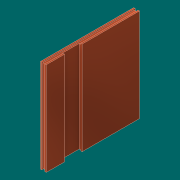
# Autodesk Inventor part: sides
Saved by Autodesk Inventor 2016 (Build 200138000, 138)
## iProperties
Created: 2015-10-13
Part Number: sides
Material: PC/ABS Plastic
Document SubType Name: Modeling
Designer: Sawaiz
Density: 0.357273 g/cm^3
Appearance: Copper - Polished
Author: Sawaiz
Autodesk Inventor part; units mm, degrees
ref_plane "YZ Plane" through (0, 0, 0) normal (1, 0, 0) x (0, 1, 0)
ref_plane "XZ Plane" through (0, 0, 0) normal (0, 1, 0) x (-1, 0, 0)
ref_plane "XY Plane" through (0, 0, 0) normal (0, 0, 1) x (1, 0, 0)
sketch "Sketch1" plane through (0, 0, 0) normal (0, 1, 0) x (-1, 0, 0)
  line L0 (-50.8, 50.8) -> (50.8, 50.8)
  line L1 (50.8, 50.8) -> (50.8, -50.8)
  line L2 (50.8, -50.8) -> (-50.8, -50.8)
  line L3 (-50.8, -50.8) -> (-50.8, 50.8)
  line L4 (-50.8, 50.8) -> (50.8, -50.8) construction
  line L5 (50.8, 50.8) -> (-50.8, -50.8) construction
  point P0 (0, 0)
  dimension "d0" = 101.6
  dimension "d1" = 101.6
  constraints: 12 end point, 2 midpoint, 2 parallel, 1 horizontal, 1 perpendicular
  measures "d0" distance of L1.end L2.end
  measures "d1" distance of L0.end L1.end
extrude "Extrusion1" add sketch "Sketch1" along normal blind 6.35
sketch "Sketch2" plane through (0, 6.35, 0) normal (0, 1, 0) x (1, 0, 0)
  line L0 (-50.8, -50.8) -> (50.8, -50.8) projected
  line L1 (50.8, -50.8) -> (50.8, 50.8) projected
  line L2 (50.8, 50.8) -> (-50.8, 50.8) projected
  line L3 (-50.8, 50.8) -> (-50.8, -50.8) projected
  line L4 (-50.8, -50.8) -> (50.8, -50.8) projected
  line L5 (30.8, 50.8) -> (11.75, 50.8)
  line L6 (11.75, 50.8) -> (11.75, -50.8)
  line L7 (11.75, -50.8) -> (30.8, -50.8)
  line L8 (30.8, -50.8) -> (30.8, 50.8)
  line L9 (30.8, 50.8) -> (11.75, -50.8) construction
  line L10 (11.75, 50.8) -> (30.8, -50.8) construction
  point P0 (0, 0)
  point P1 (21.275, 0)
  dimension "d4" = 19.05
  dimension "d5" = 20
  constraints: 12 end point, 2 collinear, 2 midpoint, 2 parallel, 1 horizontal, 1 perpendicular
  measures "d4" distance between parallel lines of L6 L8
  measures "d5" distance between parallel lines of L1 L8
extrude "Extrusion2" cut sketch "Sketch2" against normal blind 3.175 contours L6 L2 L8 L0
sketch "Sketch5" plane through (50.8, 0, 50.8) normal (1, 0, 0) x (0, 0, -1)
  line L0 (101.6, 0) -> (0, 0) projected
  line L1 (101.6, 0) -> (101.6, 6.35) projected
  line L2 (0, 6.35) -> (101.6, 6.35) projected
  line L3 (0, 0) -> (0, 6.35) projected
  line L4 (0, 0) -> (0, 6.35) projected
  line L5 (0, 3.175) -> (101.6, 3.175)
  line L6 (101.6, 1.5875) -> (0, 1.5875)
  line L7 (0, 1.5875) -> (0, 4.7625)
  line L8 (0, 4.7625) -> (101.6, 4.7625)
  line L9 (101.6, 4.7625) -> (101.6, 1.5875)
  line L10 (0, 3.175) -> (101.6, 3.175) projected
  line L11 (101.6, 1.5875) -> (0, 4.7625) construction
  line L12 (0, 1.5875) -> (101.6, 4.7625) construction
  point P0 (50.8, 0)
  point P1 (50.8, 3.175)
  point P2 (6.35, 3.175)
  point P3 (95.25, 3.175)
  dimension "d34" = 3.175
  constraints: 14 end point, 5 midpoint, 2 parallel, 1 horizontal, 1 perpendicular, 1 point on line
  measures "d34" distance between parallel lines of L8 L6
extrude "Extrusion3" cut sketch "Sketch5" against normal blind 0.9525 contours L6 L3 L5 L1 | L5 L3 L8 L1
mirror "Mirror3" about plane through (0, 0, 0) normal (1, 0, 0) of "Extrusion3"
sketch "Sketch6" plane through (-50.8, 0, 50.8) normal (0, 0, 1) x (1, 0, 0)
  line L0 (0, 4.7625) -> (0.9525, 4.7625) projected
  line L1 (0.9525, 4.7625) -> (0.9525, 1.5875) projected
  line L2 (0.9525, 1.5875) -> (0, 1.5875) projected
  line L3 (0, 0) -> (0, 1.5875) projected
  line L4 (101.6, 0) -> (0, 0) projected
  line L5 (101.6, 0) -> (101.6, 1.5875) projected
  line L6 (101.6, 1.5875) -> (100.6475, 1.5875) projected
  line L7 (100.6475, 1.5875) -> (100.6475, 4.7625) projected
  line L8 (100.6475, 4.7625) -> (101.6, 4.7625) projected
  line L9 (101.6, 4.7625) -> (101.6, 6.35) projected
  line L10 (0, 6.35) -> (62.55, 6.35) projected
  line L11 (0, 4.7625) -> (0, 6.35) projected
  line L12 (100.6475, 1.5875) -> (0.9525, 1.5875)
  line L13 (0.9525, 1.5875) -> (0.9525, 4.7625)
  line L14 (0.9525, 4.7625) -> (100.6475, 4.7625)
  line L15 (100.6475, 4.7625) -> (100.6475, 1.5875)
  line L16 (81.6, 6.35) -> (101.6, 6.35) projected
  line L17 (81.6, 6.35) -> (81.6, 3.175) projected
  line L18 (81.6, 3.175) -> (62.55, 3.175) projected
  line L19 (62.55, 3.175) -> (62.55, 6.35) projected
  point P0 (50.8, 0)
  constraints: 8 end point, 2 parallel, 1 horizontal, 1 perpendicular
extrude "Extrusion4" cut sketch "Sketch6" against normal blind 0.9525 contours L14 L19 L18 L17 L7 L12 L1 | L14 L17 L18 L19
mirror "Mirror4" about plane through (0, 0, 0) normal (0, 0, 1) of "Extrusion4"
equation "\"d0\" = depth"
equation "\"d1\" = depth"
equation "\"d2\" = acrylicThickness"
equation "\"d4\" = mirrorGroove"
equation "\"d5\" = aerogelThickness"
equation "\"d6\" = 0.5 * acrylicThickness"
equation "\"d34\" = oRingWidth"
equation "\"acrylicThickness\" = 6.35"
equation "\"depth\" = 101.6"
equation "\"mirrorThickness\" = 3"
equation "\"aerogelThickness\" = 20"
equation "\"height\" = 101.6"
equation "\"width\" = 101.6"
equation "\"mirrorAngle\" = 5deg"
equation "\"detectorWidth\" = 52"
equation "\"detectorHeight\" = 52"
equation "\"fresnelThickness\" = 0.1"
equation "\"focalLength\" = 76.2"
equation "\"ior\" = 1.49"
equation "\"centerThickness\" = 1.524"
equation "\"fresnelAngle\" = 90deg"
equation "\"fresnelEffectiveDiameter\" = 76.2"
equation "\"mirrorSuppourtWidth\" = 38.1"
equation "\"backGrooveBit\" = 4.8006"
equation "\"sensorHolderSensorWidth\" = 53.975"
equation "\"sensorHolderWidth\" = 88.9"
equation "\"sensorHolderSesnorHeight\" = 53.975"
equation "\"sensorHolderHeight\" = 88.9"
equation "\"sensorHolderSensorHeight\" = 53.975"
equation "\"sensorHolderORingGroove\" = 3.175"
equation "\"sensorHolderORing\" = 3.175"
equation "\"sensorHolderFlushORingID\" = 304.8"
equation "\"sensorHolderFlushORing\" = 3.175"
equation "\"frontBackORingID\" = 419.1"
equation "\"oRingWidth\" = 3.175"
equation "\"sensorHolderORingID\" = 203.2"
equation "\"topBottomHorizontalMirrorGroove\" = 12.7"
equation "\"backMirrorGroove\" = 6.35"
equation "\"mirrorGroove\" = 19.05"
equation "\"fresnelChamfer\" = 6.35"
equation "\"mirrorGrooveFillet\" = 6.35"
equation "\"mirrorGrooveDrill\" = 6.35"
equation "\"mirrorGrooveMill\" = 3.175"
equation "\"fresnelMirrorChamfer\" = 6.35"
equation "\"detectorOpeningHeight\" = 76.2"
equation "\"detectorOpeningWidth\" = 76.2"
body "Solid1"
